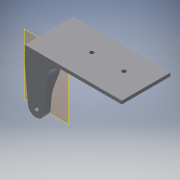
# Autodesk Inventor part: pivot2
Saved by Autodesk Inventor 2019 (Build 230136000, 136)
## iProperties
Created: 2019-02-28
Part Number: pivot2
Material: Generic
Document SubType Name: Modeling
Designer: erwin
Density: 1 g/cm^3
Appearance: Default
Author: erwin
Autodesk Inventor part; units mm, degrees
ref_plane "YZ Plane" through (0, 0, 0) normal (1, 0, 0) x (0, 1, 0)
ref_plane "XZ Plane" through (0, 0, 0) normal (0, 1, 0) x (-1, 0, 0)
ref_plane "XY Plane" through (0, 0, 0) normal (0, 0, 1) x (1, 0, 0)
ref_plane "Work Plane1" through (0, 0, 0) normal (0, 0, 1) x (1, 0, 0)
sketch "Sketch1" plane through (0, 0, 0) normal (0, 0, 1) x (1, 0, 0)
  circle A0 centre (0, 28) radius 4 projected
  circle A1 centre (0, 28) radius 3.5
  point P0 (0, 0)
  dimension "d0" = 0.5
  constraints: 1 centre point
  measures "d0" radial gap between concentric circles of A0 A1
extrude "Extrusion1" add sketch "Sketch1" against normal blind 12 contours A1
sketch "Sketch2" plane through (0, 28, 0) normal (0, 0, 1) x (1, 0, 0)
  circle A0 centre (0, 0) radius 4 projected
  circle A1 centre (0, 0) radius 5
  point P0 (0, -28)
  dimension "d3" = 1
  constraints: 1 centre point
  measures "d3" radial gap between concentric circles of A0 A1
extrude "Extrusion2" add sketch "Sketch2" along normal blind 2 contours A0 | A1
ref_plane "Work Plane2" through (0, 28, -10) normal (0, 0, -1) x (-1, 0, 0)
split body "Split1" result two bodies by plane through (0, 28, -10) normal (0, 0, -1) first body at (2.9903, 27.7586, -11.3333)
offset faces "Size1" outward 0.7 bodies 2 faces at (3.4887, 27.7184, -11.3333)
fillet "Fillet1" radius 1 2 edges at (-4.2, 28, -12) (-4.2, 28, -10)
sketch "Sketch3" plane through (0, 28, -10) normal (0, 0, -1) x (-1, 0, 0)
  line L0 (-1.25, 5) -> (1.25, 5)
  line L1 (1.25, 5) -> (1.25, -5)
  line L2 (1.25, -5) -> (-1.25, -5)
  line L3 (-1.25, -5) -> (-1.25, 5)
  line L4 (-1.25, 5) -> (1.25, -5) construction
  line L5 (1.25, 5) -> (-1.25, -5) construction
  point P0 (0, -28)
  point P1 (0, 0)
  dimension "d9" = 2.5
  dimension "d10" = 10
  constraints: 12 end point, 2 midpoint, 2 parallel, 1 horizontal, 1 perpendicular
  measures "d9" distance of L1.end L2.end
  measures "d10" distance of L0.end L1.end
extrude "Extrusion3" cut sketch "Sketch3" along normal mid plane 10 bodies 2 3
move faces "Move1" translate (0, 0, 3) faces at (1.2959, 29.5041, 2)
sketch "Sketch4" plane through (0, 28, 5) normal (0, 0, 1) x (1, 0, 0)
  circle A0 centre (0, 0) radius 5 projected
  circle A1 centre (0, 0) radius 7
  line L0 (7, 0) -> (-7, 0)
  line L1 (-7, 0) -> (-7, 7.5)
  line L2 (-7, 7.5) -> (7, 7.5)
  line L3 (7, 7.5) -> (7, 0)
  point P0 (0, -28)
  dimension "d16" = 2
  dimension "d17" = 14
  dimension "d18" = 7.5
  constraints: 8 end point, 2 parallel, 1 horizontal, 1 horizontal alignment, 1 perpendicular, 2 other
  measures "d17" distance of L1.end L2.end
  measures "d18" distance of L0.end L1.end
extrude "Extrusion4" add sketch "Sketch4" against normal blind 4 and the other way blind 1 bodies 3
sketch "Sketch5" plane through (-7, 35.5, 1) normal (0, 1, 0) x (1, 0, 0)
  line L0 (14, -5) -> (14, 0) projected
  line L1 (0, 0) -> (14, 0) projected
  line L2 (0, -5) -> (0, 0) projected
  line L3 (14, -5) -> (0, -5) projected
  line L4 (0, -5) -> (0, 0) projected
  line L5 (0, -5) -> (60, -5)
  line L6 (60, -5) -> (60, 22)
  line L7 (60, 22) -> (0, 22)
  line L8 (0, 22) -> (0, -5)
  point P0 (7, 1)
  dimension "d23" = 60
  dimension "d24" = 27
  constraints: 8 end point, 2 parallel, 1 horizontal, 1 perpendicular
  measures "d23" distance of L7.end L6.end
  measures "d24" distance of L6.end L5.end
extrude "Extrusion5" add sketch "Sketch5" along normal blind 2 bodies 3
fillet "Fillet2" radius 10 1 edges at (7, 35.5, 3.5)
sketch "Sketch6" plane through (-7, 37.5, 1) normal (0, 1, 0) x (1, 0, 0)
  line L0 (0, 22) -> (0, -5) construction
  line L1 (0, 8.5) -> (60, 8.5) construction
  line L2 (60, -5) -> (60, 22) construction
  line L3 (30, 8.5) -> (30, 22) construction
  line L4 (60, 22) -> (0, 22) construction
  line L5 (0, 22) -> (30, 22) construction
  line L6 (15, 22) -> (15, 8.5) construction
  line L7 (30, 22) -> (60, 22) construction
  line L8 (45, 22) -> (45, 8.5) construction
  point P0 (7, 1)
  constraints: 12 end point, 6 midpoint, 3 perpendicular, 2 coincident, 2 point on line, 1 collinear
hole "Hole1" at (8, 37.5, -7.5) at (38, 37.5, -7.5) direction (0, -1, 0) diameter 2.5 end through all both bodies 3
move faces "Move2" translate (0, 0, 3) faces at (-2.1512, 31.5846, 6)
sketch "Sketch7" plane through (16.8152, 35.5, 9) normal (0, 0, 1) x (1, 0, 0)
  arc A0 (-23.8152, -7.5) -> (-9.8913, -8.5294) centre (-16.8152, -7.5) ccw projected
  arc A1 (0, 0) -> (-9.8913, -8.5294) centre (0, -10) ccw projected
  line L0 (0, 0) -> (36.1848, 0) projected
  line L1 (36.1848, 0) -> (36.1848, 2) projected
  line L2 (-23.8152, 2) -> (36.1848, 2) projected
  line L3 (-23.8152, -7.5) -> (-23.8152, 2) projected
  line L4 (-1.8152, -34.5) -> (-31.8152, -34.5) projected
  circle A2 centre (-16.8152, -7.5) radius 7
  line L5 (-16.8152, -7.5) -> (-16.8152, -28.5)
  circle A3 centre (-16.8152, -28.5) radius 5
  arc A4 (-23.8152, -7.5) -> (-9.8913, -8.5294) centre (-16.8152, -7.5) ccw projected
  line L6 (-23.8152, -7.5) -> (-21.8152, -28.5)
  line L7 (-11.8152, -28.5) -> (-9.8913, -8.5294)
  point P0 (-16.8152, -35.5)
  dimension "d38" = 10
  dimension "d39" = 21
  constraints: 6 end point, 3 point on circle, 2 coincident, 1 centre point, 1 vertical, 3 other
  measures "d38" diameter of A3
  measures "d39" distance of L5.start L5.end
extrude "Extrusion6" add sketch "Sketch7" against normal blind 4 contours L3 L2 L1 L0 A1 A2 | A2 A0 L6 | A0 L5 A3 L6 | A0 L7 A3 L5 | A3 bodies 3
move faces "Move3" translate (10, 0, 0) faces at (8.1006, 36.8333, -6.2541)
sketch "Sketch8" plane through (16.8152, 35.5, 5) normal (0, 0, -1) x (-1, 0, 0)
  arc A0 (11.8152, -28.5) -> (21.8152, -28.5) centre (16.8152, -28.5) ccw projected
  point P0 (16.8152, -35.5)
  constraints: 1 coincident
hole "Hole2" at (0, 7, 5) direction (0, 0, 1) diameter 3 end through all both bodies 3
fillet "Fillet3" radius 10 1 edges at (0.1481, 21.0016, 5)
fillet "Fillet4" radius 1 2 edges at (0.3728, 35.5, 1) (12.2804, 35.5, 1)
body "Solid2"
body "Solid3"
